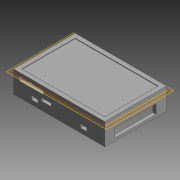
# Autodesk Inventor part: Boden
Saved by Autodesk Inventor 2014 (Build 180170000, 170)
## iProperties
Created: 2016-07-15
Part Number: Boden
Material: Generisch
Document SubType Name: Modeling
Designer: cem
Density: 1 g/cm^3
Appearance: Vorgabe
Author: cem
Autodesk Inventor part; units mm, degrees
ref_plane "YZ Plane" through (0, 0, 0) normal (1, 0, 0) x (0, 1, 0)
ref_plane "XZ Plane" through (0, 0, 0) normal (0, 1, 0) x (-1, 0, 0)
ref_plane "XY Plane" through (0, 0, 0) normal (0, 0, 1) x (1, 0, 0)
ref_plane "Arbeitsebene1" through (0, 0, 2) normal (0, 0, 1) x (1, 0, 0)
sketch "Skizze1" plane through (0, 0, 2) normal (0, 0, 1) x (1, 0, 0)
  line L0 (-18.7, 2.8) -> (-4.7, 2.8) projected
  line L1 (-4.7, 2.8) -> (-4.7, -12.4) projected
  line L2 (-4.7, -12.4) -> (-7.2, -12.4) projected
  line L3 (-7.2, -12.4) -> (-7.2, -11.4) projected
  line L4 (-7.2, -11.4) -> (-18.7, -11.4) projected
  line L5 (-18.7, -11.4) -> (-18.7, 2.8) projected
  line L6 (20, 13) -> (-20, 13) projected
  line L7 (-20, 13) -> (-20, -13) projected
  line L8 (-20, -13) -> (20, -13) projected
  line L9 (20, -13) -> (20, 13) projected
  line L10 (-21.6, 14.6) -> (21.6, 14.6)
  line L11 (21.6, 14.6) -> (21.6, -14.6)
  line L12 (21.6, -14.6) -> (-21.6, -14.6)
  line L13 (-21.6, -14.6) -> (-21.6, 14.6)
  point P0 (0, 0)
  dimension "d0" = 1.6
  constraints: 8 end point, 3 other
  measures "d0" distance between parallel lines of L10 L6
extrude "Boden" add sketch "Skizze1" along normal blind 1.5 contours L0 L1 L2 L3 L4 L5 | L9 L8 L7 L6 | L10 L11 L12 L13
ref_plane "Arbeitsebene2" through (-17.7, 4.9, -6.8) normal (0, 0, -1) x (-1, 0, 0)
sketch "Skizze2" plane through (0, 0, 2) normal (0, 0, -1) x (-1, 0, 0)
  line L0 (21.6, 14.6) -> (-21.6, 14.6) projected
  line L1 (-21.6, 14.6) -> (-21.6, -14.6) projected
  line L2 (-21.6, -14.6) -> (21.6, -14.6) projected
  line L3 (21.6, -14.6) -> (21.6, 14.6) projected
  line L4 (-20.1, -13.1) -> (-20.1, 13.1)
  line L5 (-20.1, 13.1) -> (20.1, 13.1)
  line L6 (20.1, 13.1) -> (20.1, -13.1)
  line L7 (20.1, -13.1) -> (-20.1, -13.1)
  point P0 (0, 0)
  dimension "d3" = 1.5
  constraints: 8 end point, 3 other
  measures "d3" distance between parallel lines of L4 L1
extrude "Wand" add sketch "Skizze2" along normal up to surface (8.8 mm away)
sketch "Skizze7" plane through (0, 0, 2) normal (0, 0, -1) x (-1, 0, 0)
  line L0 (-20.1, -13.1) -> (20.1, -13.1) projected
  line L1 (20.1, -13.1) -> (20.1, 13.1) projected
  line L2 (20.1, 13.1) -> (-20.1, 13.1) projected
  line L3 (-20.1, 13.1) -> (-20.1, -13.1) projected
  line L4 (-15.1, -1.1) -> (-13.1, -1.1)
  line L5 (-13.1, -1.1) -> (-13.1, -11.1)
  line L6 (-13.1, -11.1) -> (-15.1, -11.1)
  line L7 (-15.1, -11.1) -> (-15.1, -1.1)
  line L8 (18.1, 9.1) -> (-1.9, 9.1)
  line L9 (-1.9, 9.1) -> (-1.9, 7.1)
  line L10 (-1.9, 7.1) -> (18.1, 7.1)
  line L11 (18.1, 7.1) -> (18.1, 9.1)
  line L12 (-5.1, -0.9) -> (-3.1, -0.9)
  line L13 (-3.1, -0.9) -> (-3.1, -10.9)
  line L14 (-3.1, -10.9) -> (-5.1, -10.9)
  line L15 (-5.1, -10.9) -> (-5.1, -0.9)
  point P0 (0, 0)
  dimension "d16" = 2
  dimension "d17" = 4
  dimension "d18" = 2
  dimension "d19" = 20
  dimension "d20" = 2
  dimension "d21" = 10
  dimension "d22" = 8
  dimension "d23" = 5
  constraints: 24 end point, 6 parallel, 3 equal length, 3 horizontal, 3 perpendicular
  measures "d16" distance between parallel lines of L5 L7
  measures "d17" distance between parallel lines of L2 L8
  measures "d18" distance between parallel lines of L0 L6
  measures "d19" distance between parallel lines of L11 L9
  measures "d20" distance between parallel lines of L1 L11
  measures "d21" distance between parallel lines of L6 L4
  measures "d22" distance between parallel lines of L15 L5
  measures "d23" distance between parallel lines of L7 L3
extrude "Auflage" add sketch "Skizze7" along normal blind 1.8 contours L4 L5 L6 L7 | L11 L10 L9 L8 | L12 L13 L14 L15
sketch "Skizze3" plane through (21.6, 14.6, -6.8) normal (0, 0, -1) x (-1, 0, 0)
  line L0 (41.7, -1.5) -> (1.5, -1.5) projected
  line L1 (41.7, -27.7) -> (41.7, -1.5) projected
  line L2 (1.5, -27.7) -> (41.7, -27.7) projected
  line L3 (1.5, -1.5) -> (1.5, -27.7) projected
  line L4 (0, -29.2) -> (0, 0) projected
  line L5 (0.75, -28.45) -> (42.45, -28.45)
  line L6 (42.45, -28.45) -> (42.45, -0.75)
  line L7 (42.45, -0.75) -> (0.75, -0.75)
  line L8 (0.75, -0.75) -> (0.75, -28.45)
  point P0 (21.6, -14.6)
  dimension "d6" = 0.75
  constraints: 8 end point, 3 other
  measures "d6" distance between parallel lines of L4 L8
extrude "Führung" cut sketch "Skizze3" against normal blind 0.5
sketch "Skizze4" plane through (-21.6, -14.6, 3.5) normal (-1, 0, 0) x (0, 0, 1)
  line L0 (-8.8, 2.1) -> (-8.8, 11.1) projected
  line L1 (-5.1, 2.1) -> (-8.8, 2.1) projected
  line L2 (-5.1, 11.1) -> (-5.1, 2.1) projected
  line L3 (-5.1, 11.1) -> (-8.8, 11.1) projected
  line L4 (-5.1, 11.9) -> (-8.8, 11.9) projected
  line L5 (-5.1, 26.9) -> (-5.1, 11.9) projected
  line L6 (-5.1, 26.9) -> (-8.8, 26.9) projected
  line L7 (-8.8, 11.9) -> (-8.8, 26.9) projected
  line L8 (-9.1, 27.2) -> (-4.8, 27.2)
  line L9 (-4.8, 27.2) -> (-4.8, 1.8)
  line L10 (-4.8, 1.8) -> (-9.1, 1.8)
  line L11 (-9.1, 1.8) -> (-9.1, 27.2)
  point P0 (-3.5, 14.6)
  dimension "d9" = 0.3
  dimension "d10" = 0.3
  dimension "d11" = 0.3
  dimension "d12" = 0.3
  constraints: 8 end point, 2 parallel, 1 horizontal, 1 perpendicular
  measures "d9" distance between parallel lines of L7 L11
  measures "d10" distance between parallel lines of L9 L5
  measures "d11" distance between parallel lines of L6 L8
  measures "d12" distance between parallel lines of L1 L10
extrude "Stecker A" cut sketch "Skizze4" against normal up to surface (1.5 mm away) contours L0 L3 L2 L1 | L4 L7 L6 L5 | L8 L9 L10 L11
ref_plane "Arbeitsebene3" through (-4.7, -4.8, 1.95) normal (0, 0, 1) x (1, 0, 0)
sketch "Skizze6" plane through (-21.6, -14.6, 3.5) normal (0, -1, 0) x (1, 0, 0)
  line L0 (2.8, -1.55) -> (14.3, -1.55) projected
  line L1 (2.8, -3.5) -> (2.8, -1.55) projected
  line L2 (14.1, -1.7) -> (3, -1.7) projected
  line L3 (3, -1.7) -> (3, -2.7) projected
  line L4 (3, -2.7) -> (14.1, -2.7) projected
  line L5 (14.1, -2.7) -> (14.1, -1.7) projected
  line L6 (14.3, -3.5) -> (14.3, -1.55) projected
  line L7 (1.5, -3.5) -> (41.5, -3.5) projected
  line L8 (2.8, -3.5) -> (2.8, -1.55)
  line L9 (2.8, -1.55) -> (14.3, -1.55)
  line L10 (14.3, -1.55) -> (14.3, -3.5)
  line L11 (2.8, -3.5) -> (14.3, -3.5)
  point P0 (21.6, -3.5)
  dimension "d26" = 0
  constraints: 8 end point, 1 collinear, 2 other
  measures "d26" distance between parallel lines of L1 L8
extrude "SD Karte" cut sketch "Skizze6" against normal up to surface (1.5 mm away) contours L0 L6 L7 L1 | L5 L4 L3 L2
sketch "Skizze8" plane through (-21.6, -14.6, 3.5) normal (0, -1, 0) x (1, 0, 0)
  line L0 (15, -5.1) -> (15, -6.2) projected
  line L1 (16, -6.2) -> (15, -6.2) projected
  line L2 (16, -5.1) -> (16, -6.2) projected
  line L3 (17.5, -6.2) -> (16.5, -6.2) projected
  line L4 (14.5, -6.2) -> (13.5, -6.2) projected
  line L5 (13.5, -5.1) -> (13.5, -6.2) projected
  line L6 (14.5, -5.1) -> (14.5, -6.2) projected
  line L7 (17.5, -5.1) -> (17.5, -6.2) projected
  line L8 (16.5, -5.1) -> (16.5, -6.2) projected
  line L9 (13.2, -5.1) -> (17.8, -5.1)
  line L10 (17.8, -5.1) -> (17.8, -6.5)
  line L11 (17.8, -6.5) -> (13.2, -6.5)
  line L12 (13.2, -6.5) -> (13.2, -5.1)
  line L13 (41.5, -5.1) -> (1.5, -5.1) projected
  point P0 (21.6, -3.5)
  dimension "d31" = 0.3
  dimension "d32" = 0.3
  dimension "d33" = 0.3
  constraints: 8 end point, 2 parallel, 1 collinear, 1 horizontal, 1 perpendicular
  measures "d31" distance between parallel lines of L5 L12
  measures "d32" distance between parallel lines of L4 L11
  measures "d33" distance between parallel lines of L7 L10
extrude "LED" cut sketch "Skizze8" against normal up to surface (1.5 mm away)
sketch "Skizze9" plane through (21.6, -14.6, 3.5) normal (1, 0, 0) x (0, 0, -1)
  line L0 (8.8, 23.9) -> (8.8, 14.9) projected
  line L1 (5.1, 23.9) -> (8.8, 23.9) projected
  line L2 (5.1, 14.9) -> (5.1, 23.9) projected
  line L3 (5.1, 14.9) -> (8.8, 14.9) projected
  line L4 (5.1, 14.1) -> (8.8, 14.1) projected
  line L5 (5.1, 5.1) -> (5.1, 14.1) projected
  line L6 (5.1, 5.1) -> (8.8, 5.1) projected
  line L7 (8.8, 14.1) -> (8.8, 5.1) projected
  line L8 (4.8, 24.2) -> (9.1, 24.2)
  line L9 (9.1, 24.2) -> (9.1, 4.8)
  line L10 (9.1, 4.8) -> (4.8, 4.8)
  line L11 (4.8, 4.8) -> (4.8, 24.2)
  point P0 (3.5, 14.6)
  dimension "d36" = 0.3
  dimension "d37" = 0.3
  dimension "d38" = 0.3
  dimension "d39" = 0.3
  constraints: 8 end point, 2 parallel, 1 horizontal, 1 perpendicular
  measures "d36" distance between parallel lines of L2 L11
  measures "d37" distance between parallel lines of L9 L0
  measures "d38" distance between parallel lines of L1 L8
  measures "d39" distance between parallel lines of L10 L6
extrude "Stecker B" cut sketch "Skizze9" against normal up to surface (1.5 mm away) contours L0 L3 L2 L1 | L4 L7 L6 L5 | L8 L9 L10 L11
sketch "Skizze10" plane through (-21.6, 14.6, 3.5) normal (0, 1, 0) x (1, 0, 0)
  line L0 (28.7, 8.2) -> (20.8, 8.2) projected
  line L1 (20.8, 8.2) -> (20.8, 4.8) projected
  line L2 (20.8, 4.8) -> (28.7, 4.8) projected
  line L3 (28.7, 4.8) -> (28.7, 8.2) projected
  line L4 (20.5, 4.5) -> (20.5, 8.5)
  line L5 (20.5, 8.5) -> (29, 8.5)
  line L6 (29, 8.5) -> (29, 4.5)
  line L7 (29, 4.5) -> (20.5, 4.5)
  line L8 (43.2, 10.3) -> (0, 10.3) projected
  line L9 (20.5, 8.5) -> (20.5, 10.3)
  line L10 (29, 10.3) -> (29, 8.5)
  point P0 (21.6, 3.5)
  dimension "d42" = 0.3
  constraints: 12 end point, 2 point on line, 1 parallel, 1 perpendicular, 3 other
  measures "d42" distance between parallel lines of L1 L4
extrude "USB" cut sketch "Skizze10" against normal up to surface (1.5 mm away) contours L3 L2 L1 L0 | L4 L5 L6 L7 | L9 L8 L10 L5
fillet "Rundung1" radius 1.2 2 edges at (-1.1, 13.85, -1) (7.4, 13.85, -1)
sketch "Skizze11" plane through (-20.1, -13.1, 2) normal (0, 1, 0) x (1, 0, 0)
  line L0 (11.7, 3.6) -> (11.7, 5) projected
  line L1 (40.2, 8.3) -> (0, 8.3) projected
  line L2 (0, 0) -> (0, 8.3) projected
  line L3 (40.2, 0) -> (40.2, 8.3) projected
  line L4 (7, 6.8) -> (10, 6.8)
  line L5 (10, 6.8) -> (10, 5)
  line L6 (10, 5) -> (7, 5)
  line L7 (7, 5) -> (7, 6.8)
  line L8 (30.2, 6.8) -> (33.2, 6.8)
  line L9 (33.2, 6.8) -> (33.2, 5)
  line L10 (33.2, 5) -> (30.2, 5)
  line L11 (30.2, 5) -> (30.2, 6.8)
  point P0 (20.1, 2)
  dimension "d45" = 1.5
  dimension "d46" = 1.8
  dimension "d47" = 3
  dimension "d48" = 1.7
  dimension "d49" = 7
  dimension "d50" = 7
  dimension "d51" = 1.5
  constraints: 16 end point, 4 parallel, 2 equal length, 2 horizontal, 2 perpendicular
  measures "d45" distance between parallel lines of L1 L4
  measures "d46" distance between parallel lines of L6 L4
  measures "d47" distance between parallel lines of L5 L7
  measures "d48" distance between parallel lines of L0 L5
  measures "d49" distance between parallel lines of L2 L7
  measures "d50" distance between parallel lines of L3 L9
  measures "d51" distance between parallel lines of L1 L8
extrude "Klick1" cut sketch "Skizze11" against normal up to surface (1.5 mm away)
sketch "Skizze15" plane through (-20.1, 13.1, 2) normal (0, -1, 0) x (1, 0, 0)
  line L0 (10, -6.8) -> (10, -5) projected
  line L1 (10, -5) -> (7, -5) projected
  line L2 (7, -5) -> (7, -6.8) projected
  line L3 (7, -6.8) -> (10, -6.8) projected
  line L4 (33.2, -5) -> (30.2, -5) projected
  line L5 (30.2, -5) -> (30.2, -6.8) projected
  line L6 (30.2, -6.8) -> (33.2, -6.8) projected
  line L7 (33.2, -6.8) -> (33.2, -5) projected
  line L8 (16.3, -3.6) -> (11.7, -3.6) projected
  line L9 (11.7, -3.6) -> (11.7, -5) projected
  line L10 (11.7, -5) -> (16.3, -5) projected
  line L11 (16.3, -5) -> (16.3, -3.6) projected
  line L12 (1.3, -0.05) -> (1.3, -2) projected
  line L13 (1.3, -2) -> (12.8, -2) projected
  line L14 (12.8, -2) -> (12.8, -0.05) projected
  line L15 (12.8, -0.05) -> (1.3, -0.05) projected
  line L16 (40.2, -8.3) -> (0, -8.3) projected
  line L17 (0, 0) -> (0, -8.3) projected
  line L18 (40.2, 0) -> (0, 0) projected
  line L19 (40.2, 0) -> (40.2, -8.3) projected
  line L20 (33.2, -6.8) -> (30.2, -6.8)
  line L21 (30.2, -6.8) -> (30.2, -5)
  line L22 (30.2, -5) -> (33.2, -5)
  line L23 (33.2, -5) -> (33.2, -6.8)
  line L24 (10, -6.8) -> (7, -6.8)
  line L25 (7, -6.8) -> (7, -5)
  line L26 (7, -5) -> (10, -5)
  line L27 (10, -5) -> (10, -6.8)
  point P0 (20.1, -2)
  constraints: 16 end point, 4 parallel, 2 horizontal, 2 perpendicular
extrude "Klick2" cut sketch "Skizze15" against normal up to surface (1.5 mm away) contours L3 L2 L1 L0 | L7 L6 L5 L4
sketch "Skizze13" plane through (0, 0, 3.5) normal (0, 0, 1) x (1, 0, 0)
  line L0 (21.6, 14.6) -> (-21.6, 14.6) projected
  line L1 (-21.6, 14.6) -> (-21.6, -14.6) projected
  line L2 (-21.6, -14.6) -> (21.6, -14.6) projected
  line L3 (21.6, -14.6) -> (21.6, 14.6) projected
  line L4 (-19.6, -12.6) -> (-19.6, 12.6)
  line L5 (-19.6, 12.6) -> (19.6, 12.6)
  line L6 (19.6, 12.6) -> (19.6, -12.6)
  line L7 (19.6, -12.6) -> (-19.6, -12.6)
  point P0 (0, 0)
  dimension "d61" = 2
  constraints: 8 end point, 3 other
  measures "d61" distance between parallel lines of L4 L1
extrude "Aufkleber" cut sketch "Skizze13" against normal blind 0.3 contours L4 L5 L6 L7
